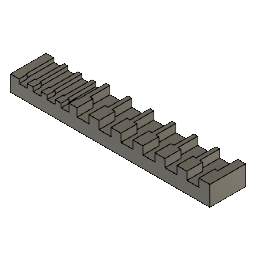
CClampRack2and3in v15 (Autodesk Fusion 360 design; units mm, degrees)
Autodesk Fusion 360 part; units mm, degrees
sketch "Sketch1" plane through (0, 0, 0) normal (0, 0, 1) x (1, 0, 0)
  line L0 (0, 57.15) -> (0, 0)
  line L1 (101.6, 57.15) -> (130.175, 57.15)
  line L2 (130.175, 57.15) -> (130.175, 25.4)
  line L3 (130.175, 25.4) -> (101.6, 25.4)
  line L4 (101.6, 25.4) -> (101.6, 57.15)
  line L5 (115.8875, 25.4) -> (115.8875, 0) construction
  line L6 (106.3625, 25.4) -> (106.3625, 0)
  line L7 (125.4125, 25.4) -> (125.4125, 0)
  line L8 (12.7, 57.15) -> (12.7, 12.7)
  line L9 (12.7, 12.7) -> (28.575, 12.7)
  line L10 (28.575, 12.7) -> (28.575, 57.15)
  line L11 (14.2875, 12.7) -> (14.2875, 0)
  line L12 (26.9875, 12.7) -> (26.9875, 0)
  line L13 (12.7, 57.15) -> (28.575, 57.15)
  line L14 (14.2875, 0) -> (26.9875, 0)
  line L15 (106.3625, 0) -> (125.4125, 0)
  line L16 (36.5125, 0) -> (49.2125, 0)
  line L17 (34.925, 57.15) -> (50.8, 57.15)
  line L18 (49.2125, 12.7) -> (49.2125, 0)
  line L19 (34.925, 57.15) -> (34.925, 12.7)
  line L20 (36.5125, 12.7) -> (36.5125, 0)
  line L21 (34.925, 12.7) -> (50.8, 12.7)
  line L22 (50.8, 12.7) -> (50.8, 57.15)
  line L23 (58.7375, 0) -> (71.4375, 0)
  line L24 (57.15, 57.15) -> (73.025, 57.15)
  line L25 (71.4375, 12.7) -> (71.4375, 0)
  line L26 (57.15, 57.15) -> (57.15, 12.7)
  line L27 (58.7375, 12.7) -> (58.7375, 0)
  line L28 (57.15, 12.7) -> (73.025, 12.7)
  line L29 (73.025, 12.7) -> (73.025, 57.15)
  line L30 (80.9625, 0) -> (93.6625, 0)
  line L31 (79.375, 57.15) -> (95.25, 57.15)
  line L32 (93.6625, 12.7) -> (93.6625, 0)
  line L33 (79.375, 57.15) -> (79.375, 12.7)
  line L34 (80.9625, 12.7) -> (80.9625, 0)
  line L35 (79.375, 12.7) -> (95.25, 12.7)
  line L36 (95.25, 12.7) -> (95.25, 57.15)
  line L37 (141.2875, 25.4) -> (141.2875, 0)
  line L38 (136.525, 57.15) -> (165.1, 57.15)
  line L39 (150.8125, 25.4) -> (150.8125, 0) construction
  line L40 (136.525, 25.4) -> (136.525, 57.15)
  line L41 (165.1, 25.4) -> (136.525, 25.4)
  line L42 (165.1, 57.15) -> (165.1, 25.4)
  line L43 (160.3375, 25.4) -> (160.3375, 0)
  line L44 (141.2875, 0) -> (160.3375, 0)
  line L45 (176.2125, 25.4) -> (176.2125, 0)
  line L46 (171.45, 57.15) -> (200.025, 57.15)
  line L47 (185.7375, 25.4) -> (185.7375, 0) construction
  line L48 (171.45, 25.4) -> (171.45, 57.15)
  line L49 (200.025, 25.4) -> (171.45, 25.4)
  line L50 (200.025, 57.15) -> (200.025, 25.4)
  line L51 (195.2625, 25.4) -> (195.2625, 0)
  line L52 (176.2125, 0) -> (195.2625, 0)
  line L53 (211.1375, 25.4) -> (211.1375, 0)
  line L54 (206.375, 57.15) -> (234.95, 57.15)
  line L55 (220.6625, 25.4) -> (220.6625, 0) construction
  line L56 (206.375, 25.4) -> (206.375, 57.15)
  line L57 (234.95, 25.4) -> (206.375, 25.4)
  line L58 (234.95, 57.15) -> (234.95, 25.4)
  line L59 (230.1875, 25.4) -> (230.1875, 0)
  line L60 (211.1375, 0) -> (230.1875, 0)
  line L61 (317.5, 57.15) -> (317.5, 0)
  line L62 (317.5, 0) -> (0, 0)
  line L63 (317.5, 57.15) -> (0, 57.15)
  line L64 (265.1125, 25.4) -> (265.1125, 0)
  line L65 (241.3, 57.15) -> (269.875, 57.15)
  line L66 (255.5875, 25.4) -> (255.5875, 0) construction
  line L67 (246.0625, 25.4) -> (246.0625, 0)
  line L68 (269.875, 25.4) -> (241.3, 25.4)
  line L69 (246.0625, 0) -> (265.1125, 0)
  line L70 (269.875, 57.15) -> (269.875, 25.4)
  line L71 (241.3, 25.4) -> (241.3, 57.15)
  line L72 (300.0375, 25.4) -> (300.0375, 0)
  line L73 (276.225, 57.15) -> (304.8, 57.15)
  line L74 (290.5125, 25.4) -> (290.5125, 0) construction
  line L75 (280.9875, 25.4) -> (280.9875, 0)
  line L76 (304.8, 25.4) -> (276.225, 25.4)
  line L77 (280.9875, 0) -> (300.0375, 0)
  line L78 (304.8, 57.15) -> (304.8, 25.4)
  line L79 (276.225, 25.4) -> (276.225, 57.15)
  dimension "d2" = 57.15
  dimension "d4" = 28.575
  dimension "d6" = 9.525
  dimension "d7" = 9.525
  dimension "d21" = 15.875
  dimension "d23" = 12.7
  dimension "d24" = 1.5875
  dimension "d25" = 15.875
  dimension "d26" = 12.7
  dimension "d27" = 1.5875
  dimension "d28" = 15.875
  dimension "d29" = 12.7
  dimension "d30" = 1.5875
  dimension "d31" = 15.875
  dimension "d32" = 12.7
  dimension "d33" = 1.5875
  dimension "d34" = 6.35
  dimension "d35" = 6.35
  dimension "d36" = 6.35
  dimension "d37" = 12.7
  dimension "d38" = 6.35
  dimension "d39" = 31.75
  dimension "d40" = 28.575
  dimension "d41" = 9.525
  dimension "d42" = 9.525
  dimension "d43" = 31.75
  dimension "d44" = 28.575
  dimension "d45" = 9.525
  dimension "d46" = 9.525
  dimension "d47" = 31.75
  dimension "d48" = 28.575
  dimension "d49" = 9.525
  dimension "d50" = 9.525
  dimension "d51" = 31.75
  dimension "d52" = 6.35
  dimension "d53" = 6.35
  dimension "d54" = 6.35
  dimension "d56" = 28.575
  dimension "d57" = 9.525
  dimension "d58" = 9.525
  dimension "d59" = 31.75
  dimension "d60" = 28.575
  dimension "d61" = 9.525
  dimension "d62" = 9.525
  dimension "d63" = 31.75
  dimension "d64" = 6.35
  dimension "d65" = 6.35
  dimension "d66" = 12.7
  measures "d6" distance of L5 L6
  measures "d7" distance of L5 L7
  measures "d21" distance of L8 L10
  measures "d23" distance of L11 L12
  measures "d24" distance of L8 L11
  measures "d25" distance of L19 L22
  measures "d26" distance of L18 L20
  measures "d27" distance of L19 L20
  measures "d28" distance of L26 L29
  measures "d29" distance of L25 L27
  measures "d30" distance of L26 L27
  measures "d31" distance of L33 L36
  measures "d32" distance of L32 L34
  measures "d33" distance of L33 L34
  measures "d34" distance of L10 L19
  measures "d35" distance of L22 L26
  measures "d36" distance of L29 L33
  measures "d37" distance of L0 L8
  measures "d38" distance of L4 L36
  measures "d41" distance of L37 L39
  measures "d42" distance of L39 L43
  measures "d45" distance of L45 L47
  measures "d46" distance of L47 L51
  measures "d49" distance of L53 L55
  measures "d50" distance of L55 L59
  measures "d52" distance of L2 L40
  measures "d53" distance of L42 L48
  measures "d54" distance of L50 L56
  measures "d57" distance of L66 L67
  measures "d58" distance of L64 L66
  measures "d61" distance of L74 L75
  measures "d62" distance of L72 L74
  measures "d64" distance of L58 L71
  measures "d65" distance of L70 L79
  measures "d66" distance of L61 L78
extrude "Extrude3" add sketch "Sketch1" against normal blind 31.75
extrude "Extrude6" cut sketch "Sketch1" against normal blind 12.7 contours L1 L2 L3 L4 L63 | L3 L6 L7 L15 L62 | L38 L40 L41 L42 L63 | L37 L41 L43 L44 L62 | L46 L48 L49 L50 L63 | L45 L49 L51 L52 L62 | L54 L56 L57 L58 L63 | L53 L57 L59 L60 L62 | L63 L65 L68 L70 L71 | L62 L64 L67 L68 L69 | L63 L73 L76 L78 L79 | L62 L72 L75 L76 L77
extrude "Extrude7" cut sketch "Sketch1" against normal blind 12.7 contours L8 L9 L10 L13 L63 | L9 L11 L12 L14 L62 | L17 L19 L21 L22 L63 | L16 L18 L20 L21 L62 | L24 L26 L28 L29 L63 | L23 L25 L27 L28 L62 | L31 L33 L35 L36 L63 | L30 L32 L34 L35 L62
extrude "Extrude8" cut 4 faces at (77.2583, 4.2333, 0) (55.0333, 4.2333, 0) (32.8083, 4.2333, 0) (4.2333, 23.2833, 0) along direction (0, 0, -1) blind 6.35
equation "d21 = ( 5 / 8 ) * 1 in"
equation "d24 = ( 1 / 16 ) * 1 in"
equation "d25 = ( 5 / 8 ) * 1 in"
equation "d27 = ( 1 / 16 ) * 1 in"
equation "d28 = ( 5 / 8 ) * 1 in"
equation "d30 = ( 1 / 16 ) * 1 in"
equation "d31 = ( 5 / 8 ) * 1 in"
equation "d33 = ( 1 / 16 ) * 1 in"
